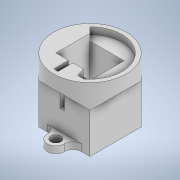
# Autodesk Inventor part: SpringPotBottom
Saved by Autodesk Inventor 2022 (Build 260153000, 153)
## iProperties
Created: 2022-04-06
Part Number: SpringPotBottom
Material: Generic
Document SubType Name: Modeling
Designer: awp
Density: 1 g/cm^3
Appearance: Default
Author: awp
Autodesk Inventor part; units mm, degrees
ref_plane "YZ Plane" through (0, 0, 0) normal (1, 0, 0) x (0, 1, 0)
ref_plane "XZ Plane" through (0, 0, 0) normal (0, 1, 0) x (-1, 0, 0)
ref_plane "XY Plane" through (0, 0, 0) normal (0, 0, 1) x (1, 0, 0)
sketch "Sketch1" plane through (0, 0, 0) normal (0, 1, 0) x (-1, 0, 0)
  line L0 (0, 0) -> (10.125, 0)
  line L1 (10.125, 0) -> (10.125, -10.125)
  line L2 (10.125, -10.125) -> (0, -10.125)
  line L3 (0, -10.125) -> (0, 0)
  line L4 (10.125, -10.125) -> (12.665, -10.125)
  line L5 (12.665, -10.125) -> (12.665, -12.665)
  line L6 (12.665, -12.665) -> (10.125, -12.665)
  line L7 (10.125, -12.665) -> (10.125, -10.125)
  line L8 (0, 0) -> (-2.54, 0)
  line L9 (-2.54, 0) -> (-2.54, 2.54)
  line L10 (-2.54, 2.54) -> (0, 2.54)
  line L11 (0, 2.54) -> (0, 0)
  line L12 (-2.54, 2.54) -> (12.665, 2.54)
  line L13 (12.665, 2.54) -> (12.665, -12.665)
  line L14 (12.665, -12.665) -> (-2.54, -12.665)
  line L15 (-2.54, -12.665) -> (-2.54, 2.54)
  dimension "d0" = 10.125
  dimension "d1" = 10.125
  dimension "d2" = 2.54
  dimension "d3" = 2.54
  dimension "d4" = 2.54
  dimension "d5" = 2.54
  constraints: 32 end point, 8 parallel, 4 horizontal, 4 perpendicular
  measures "d0" distance of L1.end L2.end
  measures "d1" distance of L0.end L1.end
  measures "d2" distance of L5.end L6.end
  measures "d3" distance of L4.end L5.end
  measures "d4" distance of L9.end L10.end
  measures "d5" distance of L8.end L9.end
extrude "Extrusion1" add sketch "Sketch1" along normal blind 8 contours L11 L12 L13 L4 L1 L0 | L3 L2 L7 L14 L15 L8 | L8 L9 L10 L11 | L4 L5 L6 L7
sketch "Sketch2" plane through (0, 8, 0) normal (0, 1, 0) x (1, 0, 0)
  line L0 (2.54, -2.54) -> (-5.0625, -2.54)
  line L1 (-12.665, -2.54) -> (2.54, -2.54) projected
  line L2 (-5.0625, -2.54) -> (-5.0625, 0)
  line L3 (0, 0) -> (-10.125, 0) projected
  line L4 (-5.0625, -2.54) -> (-6.3325, -2.54)
  line L5 (-6.3325, -2.54) -> (-6.3325, 0)
  line L6 (-6.3325, 0) -> (-5.0625, 0)
  line L7 (-12.665, 12.665) -> (-12.665, -2.54) projected
  line L8 (-12.665, -2.54) -> (2.54, -2.54) projected
  line L9 (2.54, -2.54) -> (2.54, 12.665) projected
  line L10 (2.54, 12.665) -> (-12.665, 12.665) projected
  line L11 (-10.125, 10.125) -> (0, 10.125) projected
  line L12 (0, 10.125) -> (0, 0) projected
  line L13 (0, 0) -> (-10.125, 0) projected
  line L14 (-10.125, 0) -> (-10.125, 10.125) projected
  point P0 (-6.3325, 0)
  point P1 (-10.125, 0)
  dimension "d8" = 1.27
  constraints: 10 end point, 2 midpoint, 2 perpendicular, 1 point on line
  measures "d8" distance of L0.end L4.end
extrude "Extrusion2" add sketch "Sketch2" along normal blind 11 contours L0 L2 L3 L12 L11 L14 L5 L1 L7 L10 L9
sketch "Sketch3" plane through (0, 19, 0) normal (0, 1, 0) x (1, 0, 0)
  line L0 (2.54, -2.54) -> (2.54, 12.665)
  line L1 (2.54, -2.54) -> (0, 0)
  line L2 (-10.125, 10.125) -> (0, 10.125)
  line L3 (2.54, 12.665) -> (0, 10.125)
  line L4 (0, 10.125) -> (0, 0)
  line L5 (2.54, 12.665) -> (-12.665, 12.665)
  line L6 (-12.665, -2.54) -> (2.54, -2.54)
  line L7 (2.54, 12.665) -> (2.54, -2.54)
  line L8 (-0.820593, 10.125) -> (-0.820593, 12.665)
  line L9 (-10.125, 10.125) -> (-12.665, 12.665)
  line L10 (0, 0) -> (-10.125, 0)
  line L11 (-1.948928, 0) -> (-1.136692, -2.54)
  constraints: 14 end point, 4 point on line, 2 perpendicular
extrude "Extrusion3" cut sketch "Sketch3" against normal blind 2
sketch "Sketch4" plane through (0, 19, 0) normal (0, 1, 0) x (1, 0, 0)
  line L0 (-12.665, 12.665) -> (-12.665, -2.54)
  line L1 (-12.665, -2.54) -> (-6.3325, -2.54)
  line L2 (-6.3325, -2.54) -> (-6.3325, 0)
  line L3 (-6.3325, 0) -> (-10.125, 0)
  line L4 (-10.125, 0) -> (-10.125, 10.125)
  line L5 (-6.3325, 0) -> (-10.125, 0)
  line L6 (-5.0625, 0) -> (-5.0625, -2.54)
  line L7 (-5.0625, -2.54) -> (-1.136692, -2.54)
  line L8 (2.54, 12.665) -> (2.54, -2.54)
  line L9 (0, 0) -> (0, 10.125)
  line L10 (-12.665, 12.665) -> (-12.665, -2.54)
  line L11 (-12.665, 12.665) -> (2.54, 12.665)
  line L12 (0, 10.125) -> (-10.125, 10.125)
  line L13 (-0.820593, 10.125) -> (-0.820593, 12.665)
  line L14 (-0.820593, 10.125) -> (-0.820593, 14.880782)
  line L15 (0, 0) -> (-5.0625, 0)
  line L16 (-6.3325, 0) -> (-10.125, 0)
  line L17 (-8.310764, 0) -> (-3.174588, 0) construction
  line L18 (-5.0625, 0) -> (-5.0625, -2.54)
  line L19 (-5.0625, 0) -> (-2.5225, 0)
  line L20 (-6.3325, 0) -> (-8.8725, 0)
  line L21 (-8.8725, 0) -> (-8.8725, -4.834839)
  line L22 (-2.5225, 0) -> (-2.5225, -5.039881)
  line L23 (-2.5225, 0) -> (2.517381, 0) construction
  circle A0 centre (-5.0625, 5.0625) radius 10.751559
  line L24 (-8.8725, -4.834839) -> (-8.8725, -4.991351)
  line L25 (-2.5225, -5.039881) -> (-2.5225, -5.38472)
  line L26 (-0.820593, 14.880782) -> (-0.820593, 14.941884)
  line L27 (-10.125, 10.125) -> (-12.665, 12.665)
  line L28 (-10.125, 10.125) -> (-12.665, 12.665)
  line L29 (-6.3325, 0) -> (-6.3325, -3.581822)
  line L30 (-6.3325, 0) -> (-2.750678, 0) construction
  line L31 (-6.3325, -3.581822) -> (-6.3325, -5.613787)
  line L32 (-5.0625, 0) -> (-5.0625, -5.689059)
  line L33 (-5.0625, 0) -> (0.626559, 0) construction
  circle A1 centre (-5.0625, 5.0625) radius 9.525
  line L34 (-1.948928, 0) -> (0, 0)
  line L35 (-1.136692, -2.54) -> (-1.948928, 0)
  line L36 (2.54, -2.54) -> (-1.136692, -2.54)
  line L37 (-1.136692, -2.54) -> (-1.948928, 0)
  line L38 (-1.948928, 0) -> (-5.0625, 0)
  line L39 (-10.125, 10.125) -> (-12.665, 12.665)
  line L40 (-12.665, 12.665) -> (-12.665, -2.54)
  line L41 (-12.665, -2.54) -> (-6.3325, -2.54)
  line L42 (-6.3325, -2.54) -> (-6.3325, 0)
  line L43 (-10.125, 0) -> (-10.125, 10.125)
  point P0 (-2.5225, -2.54)
  point P1 (-8.8725, -2.54)
  point P2 (2.54, -0.675759)
  point P3 (-11.797692, 11.797692)
  point P4 (0.675759, -2.54)
  point P5 (2.54, 10.800759)
  point P6 (0.675759, 12.665)
  point P7 (-10.800759, 12.665)
  point P8 (-11.797692, 11.797692)
  point P9 (-5.0625, -4.4625)
  point P10 (-6.3325, -4.377454)
  dimension "d15" = 2.54
  dimension "d16" = 2.54
  dimension "d17" = 90
  dimension "d18" = 90
  dimension "d31" = 90
  dimension "d32" = 90
  dimension "d33" = 19.05
  constraints: 30 end point, 6 point on circle, 4 horizontal, 4 point on line, 3 perpendicular, 2 centre point, 2 vertical, 1 coincident, 1 parallel
  measures "d15" distance of L6.start L19.end
  measures "d16" distance of L2.end L20.end
  measures "d17" angle of L21 L20
  measures "d18" angle of L22 L23
  measures "d31" angle of L29 L30
  measures "d32" angle of L32 L33
  measures "d33" diameter of A1
extrude "Extrusion4" add sketch "Sketch4" against normal blind 2 contours L27 A1 L0 | A0 L26 L14 A1 L11 | L0 A1 A0 | L11 A1 L27 | A1 L27 L4 L3 L21 L1 L0 | L0 A1 | A0 L11 A1 L14 L26 | L0 A1 L1 | L1 A1 L21 L24 A0 | A0 L8 A1 | L8 A1 L11 | L1 L21 A1 | L24 L21 A1 L31 A0 | L21 L3 L2 L1 | L1 L29 L31 A1 L21 | L31 A1 L32 A0 | L8 L36 A1 | A0 L25 L22 A1 L36 | L32 A1 L22 L25 A0 | A1 L22 L7 L36 | L32 L7 L22 A1 | L6 L15 L22 L7
sketch "Sketch5" plane through (0, 17, 0) normal (0, -1, 0) x (1, 0, 0)
  line L0 (2.54, 0.675759) -> (2.54, 2.54)
  arc A0 (2.54, -10.800759) -> (2.54, 0.675759) centre (-5.0625, -5.0625) ccw
  line L1 (2.54, -12.665) -> (2.54, -10.800759)
  arc A1 (2.54, -12.665) -> (2.54, 2.54) centre (-5.0625, -5.0625) ccw
  line L2 (-12.665, 2.54) -> (-12.665, -12.665)
  arc A2 (-12.665, 2.54) -> (-12.665, -12.665) centre (-5.0625, -5.0625) ccw
  circle A3 centre (-5.0625, -5.0625) radius 10.751559
  circle A4 centre (-5.0625, -5.0625) radius 9.525
  line L3 (-10.800759, -12.665) -> (0.675759, -12.665)
  line L4 (2.54, -10.800759) -> (2.54, 0.675759)
  line L5 (-5.0625, 4.4625) -> (-5.0625, 2.54)
  line L6 (-6.3325, 2.54) -> (-6.3325, 4.377454)
  line L7 (-6.3325, 2.54) -> (-12.665, 2.54)
  line L8 (-1.136692, 2.54) -> (-5.0625, 2.54)
  line L9 (0.675759, 2.54) -> (-1.136692, 2.54)
  point P0 (0, 0)
  point P1 (-12.665, -10.800759)
  constraints: 2 centre point, 2 coincident
extrude "Extrusion5" add sketch "Sketch5" along normal blind 2 contours A4 L7 A3 L0 | L0 A1 L1 A0 | A0 L4 | L9 L8 L5 A4 | L1 A3 L2 A4 | L2 A4 A2 | A4 L3 | L2 A4 | A4 L6 L7
chamfer "Chamfer4" distance 3.14706 angle 45 3 edges at (-12.665, 15, -5.0625) (-5.0625, 15, -12.665) (2.54, 15, -5.0625)
chamfer "Chamfer5" distance 3.0734 angle 45 2 edges at (-9.4988, 15, 2.54) (-1.2613, 15, 2.54)
sketch "Sketch6" plane through (0, 0, 0) normal (0, -1, 0) x (1, 0, 0)
  line L0 (-12.665, -12.665) -> (-12.665, 2.54) projected
  line L1 (2.54, -12.665) -> (-12.665, -12.665) projected
  line L2 (2.54, 2.54) -> (2.54, -12.665) projected
  line L3 (-12.665, 2.54) -> (2.54, 2.54) projected
  line L4 (-10.125, -10.125) -> (0, -10.125) projected
  line L5 (-10.125, 0) -> (-10.125, -10.125) projected
  line L6 (0, 0) -> (-10.125, 0) projected
  line L7 (0, -10.125) -> (0, 0) projected
  line L8 (2.54, -12.665) -> (-12.665, -12.665) projected
  line L9 (-5.0625, -12.665) -> (-7.6025, -12.665)
  line L10 (-7.6025, -12.665) -> (-7.6025, -17.745)
  line L11 (-7.6025, -17.745) -> (-5.0625, -17.745)
  line L12 (-5.0625, -17.745) -> (-5.0625, -12.665)
  line L13 (-5.0625, -12.665) -> (-2.5225, -12.665)
  line L14 (-2.5225, -12.665) -> (-2.5225, -17.745)
  line L15 (-2.5225, -17.745) -> (-5.0625, -17.745)
  line L16 (-5.0625, -17.745) -> (-5.0625, -12.665)
  line L17 (-5.0625, 2.54) -> (-7.6025, 2.54)
  line L18 (-7.6025, 2.54) -> (-7.6025, 7.62)
  line L19 (-7.6025, 7.62) -> (-5.0625, 7.62)
  line L20 (-5.0625, 7.62) -> (-5.0625, 2.54)
  line L21 (-12.665, 2.54) -> (2.54, 2.54) projected
  line L22 (-5.0625, 7.62) -> (-2.5225, 7.62)
  line L23 (-2.5225, 7.62) -> (-2.5225, 2.54)
  line L24 (-2.5225, 2.54) -> (-5.0625, 2.54)
  line L25 (-5.0625, 2.54) -> (-5.0625, 7.62)
  circle A0 centre (-5.0625, -15.205) radius 1.5
  circle A1 centre (-5.0625, 5.08) radius 1.5
  point P0 (-2.5225, 2.54)
  dimension "d42" = 2.54
  dimension "d43" = 5.08
  dimension "d44" = 2.54
  dimension "d45" = 5.08
  dimension "d46" = 2.54
  dimension "d47" = 3
  dimension "d48" = 2.54
  dimension "d49" = 3
  constraints: 32 end point, 8 parallel, 4 horizontal, 4 midpoint, 4 perpendicular, 2 centre point, 2 point on line
  measures "d42" distance of L11.end L10.end
  measures "d43" distance of L10.end L9.end
  measures "d44" distance of L14.end L15.end
  measures "d45" distance of L17.end L18.end
  measures "d46" distance of L23.end L24.end
  measures "d47" diameter of A0
  measures "d48" distance of L18.end L19.end
  measures "d49" diameter of A1
extrude "Extrusion6" add sketch "Sketch6" against normal blind 2 contours L1 L12 A0 L11 L10 | L18 L19 L20 A1 L3 | L1 L14 L15 L12 A0 | L20 A1 L22 L23 L3
fillet "Fillet2" radius 2.54 8 edges at (-7.6025, 1, -17.745) (-2.5225, 1, -17.745) (-2.5225, 1, -12.665) (-7.6025, 1, -12.665) (-7.6025, 1, 2.54) (-2.5225, 1, 2.54) (-2.5225, 1, 7.62) (-7.6025, 1, 7.62)
body "Solid1"
